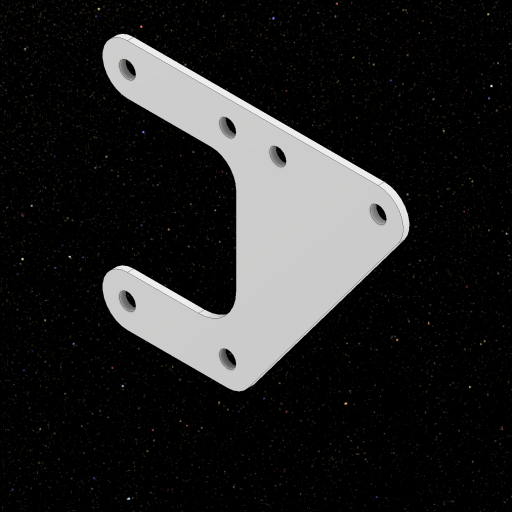
# Autodesk Inventor part: gusset
Saved by Autodesk Inventor 2024 (Build 280153000, 153)
## iProperties
Created: 2024-02-28
Part Number: gusset
Material: Acetal Resin, White
Document SubType Name: Modeling
Designer: Averey Ku
Density: 1.425 g/cm^3
Appearance: Smooth - White
Author: Averey Ku
Autodesk Inventor part; units mm, degrees
ref_plane "YZ Plane" through (0, 0, 0) normal (1, 0, 0) x (0, 1, 0)
ref_plane "XZ Plane" through (0, 0, 0) normal (0, 1, 0) x (-1, 0, 0)
ref_plane "XY Plane" through (0, 0, 0) normal (0, 0, 1) x (1, 0, 0)
sketch "main" plane through (0, 0, 0) normal (0, 0, 1) x (1, 0, 0)
  circle A0 centre (-8.7196, -23.7408) radius 2.0955
  circle A1 centre (-34.1196, -23.7408) radius 2.0955
  arc A2 (-34.1196, -17.3908) -> (-34.1196, -30.0908) centre (-34.1196, -23.7408) ccw
  arc A3 (-16.1491, -17.3908) -> (-6.6241, -7.8658) centre (-16.1491, -7.8658) ccw
  arc A4 (-8.7196, -30.0908) -> (-3.6396, -27.5508) centre (-8.7196, -23.7408) ccw
  line L0 (-16.1491, -17.3908) -> (-34.1196, -17.3908)
  line L1 (-8.7196, -30.0908) -> (-34.1196, -30.0908)
  circle A5 centre (-8.7196, 27.0592) radius 2.0955
  circle A6 centre (-34.1196, 27.0592) radius 2.0955
  arc A7 (-34.1196, 33.4092) -> (-34.1196, 20.7092) centre (-34.1196, 27.0592) ccw
  line L2 (-6.6241, 14.3592) -> (-6.6241, -7.8658)
  line L3 (-34.1196, 20.7092) -> (-12.9741, 20.7092)
  arc A8 (-6.6241, 14.3592) -> (-12.9741, 20.7092) centre (-12.9741, 14.3592) ccw
  line L4 (-3.6396, -27.5508) -> (34.4604, 23.2492)
  line L5 (-34.1196, 33.4092) -> (29.3804, 33.4092)
  line L6 (-6.6241, 20.7092) -> (15.6009, 20.7092) construction
  circle A9 centre (3.9804, 27.0592) radius 2.0955
  circle A10 centre (29.3804, 27.0592) radius 2.0955
  arc A11 (34.4604, 23.2492) -> (29.3804, 33.4092) centre (29.3804, 27.0592) ccw
  point P0 (-9.3122, 5.0882)
  dimension "d0" = 4.191
  dimension "d1" = 4.191
  dimension "d2" = 4.191
  dimension "d3" = 4.191
  dimension "d4" = 9.525
  dimension "d5" = 6.35
  measures "d0" diameter of A5
  measures "d1" diameter of A6
  measures "d2" diameter of A0
  measures "d3" diameter of A1
  measures "d4" radius of A3
  measures "d5" radius of A8
sketch "Sketch1" plane through (0, 0, 0) normal (0, 0, 1) x (1, 0, 0)
  circle A0 centre (25.4, 0) radius 2.0955
  circle A1 centre (0, 0) radius 2.0955
  arc A2 (0, 6.35) -> (0, -6.35) centre (0, 0) ccw
  arc A3 (17.9705, 6.35) -> (27.4955, 15.875) centre (17.9705, 15.875) ccw
  arc A4 (25.4, -6.35) -> (30.48, -3.81) centre (25.4, 0) ccw
  line L0 (17.9705, 6.35) -> (0, 6.35)
  line L1 (25.4, -6.35) -> (0, -6.35)
  circle A5 centre (25.4, 50.8) radius 2.0955
  circle A6 centre (0, 50.8) radius 2.0955
  arc A7 (0, 57.15) -> (0, 44.45) centre (0, 50.8) ccw
  line L2 (27.4955, 38.1) -> (27.4955, 15.875)
  line L3 (0, 44.45) -> (21.1455, 44.45)
  arc A8 (27.4955, 38.1) -> (21.1455, 44.45) centre (21.1455, 38.1) ccw
  line L4 (30.48, -3.81) -> (68.58, 46.99)
  line L5 (0, 57.15) -> (63.5, 57.15)
  line L6 (27.4955, 44.45) -> (49.7205, 44.45) construction
  circle A9 centre (38.1, 50.8) radius 2.0955
  circle A10 centre (63.5, 50.8) radius 2.0955
  arc A11 (68.58, 46.99) -> (63.5, 57.15) centre (63.5, 50.8) ccw
  constraints: 1 other
extrude "Extrusion1" add sketch "Sketch1" along normal blind 1.5875
body "Solid1"
